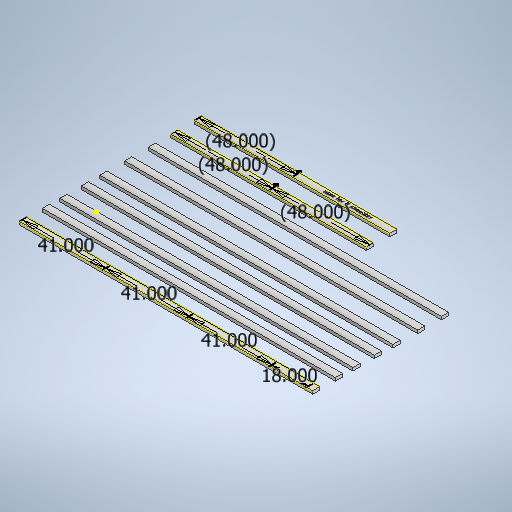
# Autodesk Inventor part: Lshoulder cuts
Saved by Autodesk Inventor 2026.1 (Build 301233000, 233)
## iProperties
Created: 2025-10-17
Part Number: Lshoulder cuts
Material: Generic
Document SubType Name: Modeling
Designer: jorda
Density: 1 g/cm^3
Appearance: Default
Author: jorda
Autodesk Inventor part; units mm, degrees
ref_plane "YZ Plane" through (0, 0, 0) normal (1, 0, 0) x (0, 1, 0)
ref_plane "XZ Plane" through (0, 0, 0) normal (0, 1, 0) x (-1, 0, 0)
ref_plane "XY Plane" through (0, 0, 0) normal (0, 0, 1) x (1, 0, 0)
sketch "Sketch1" plane through (0, 0, 0) normal (0, 1, 0) x (-1, 0, 0)
  line L0 (385.9062, 574.5992) -> (-3271.6938, 574.5992)
  line L1 (-3271.6938, 574.5992) -> (-3271.6938, 485.6992)
  line L2 (-3271.6938, 485.6992) -> (385.9062, 485.6992)
  line L3 (385.9062, 485.6992) -> (385.9062, 574.5992)
  line L4 (385.9062, 290.8577) -> (-3271.6938, 290.8577)
  line L5 (-3271.6938, 290.8577) -> (-3271.6938, 201.9577)
  line L6 (-3271.6938, 201.9577) -> (385.9062, 201.9577)
  line L7 (385.9062, 201.9577) -> (385.9062, 290.8577)
  line L8 (385.9062, 72.812) -> (-3271.6938, 72.812)
  line L9 (-3271.6938, 72.812) -> (-3271.6938, -16.088)
  line L10 (-3271.6938, -16.088) -> (385.9062, -16.088)
  line L11 (385.9062, -16.088) -> (385.9062, 72.812)
  line L12 (385.9062, -194.7435) -> (-3271.6938, -194.7435)
  line L13 (-3271.6938, -194.7435) -> (-3271.6938, -283.6435)
  line L14 (-3271.6938, -283.6435) -> (385.9062, -283.6435)
  line L15 (385.9062, -283.6435) -> (385.9062, -194.7435)
  line L16 (385.9062, -426.6687) -> (-3271.6938, -426.6687)
  line L17 (-3271.6938, -426.6687) -> (-3271.6938, -515.5687)
  line L18 (-3271.6938, -515.5687) -> (385.9062, -515.5687)
  line L19 (385.9062, -515.5687) -> (385.9062, -426.6687)
  line L20 (385.9062, -736.3666) -> (-3271.6938, -736.3666)
  line L21 (-3271.6938, -736.3666) -> (-3271.6938, -825.2666)
  line L22 (-3271.6938, -825.2666) -> (385.9062, -825.2666)
  line L23 (385.9062, -825.2666) -> (385.9062, -736.3666)
  line L24 (385.9062, -1031.6599) -> (-3271.6938, -1031.6599)
  line L25 (-3271.6938, -1031.6599) -> (-3271.6938, -1120.5599)
  line L26 (-3271.6938, -1120.5599) -> (385.9062, -1120.5599)
  line L27 (385.9062, -1120.5599) -> (385.9062, -1031.6599)
  line L28 (385.9062, -1312.5487) -> (-2052.4938, -1312.5487)
  line L29 (-2052.4938, -1312.5487) -> (-2052.4938, -1401.4487)
  line L30 (-2052.4938, -1401.4487) -> (385.9062, -1401.4487)
  line L31 (385.9062, -1401.4487) -> (385.9062, -1312.5487)
  line L32 (385.9062, -1607.8421) -> (-2052.4938, -1607.8421)
  line L33 (-2052.4938, -1607.8421) -> (-2052.4938, -1696.7421)
  line L34 (-2052.4938, -1696.7421) -> (385.9062, -1696.7421)
  line L35 (385.9062, -1696.7421) -> (385.9062, -1607.8421)
  point P0 (0, 0)
  constraints: 72 end point, 18 parallel, 9 horizontal, 9 perpendicular, 1 point on line
extrude "Extrusion1" add sketch "Sketch1" along normal blind 38.1
sketch "Sketch2" plane through (0, 38.1, 0) normal (0, 1, 0) x (1, 0, 0)
  line L0 (-385.9062, -574.5992) -> (3271.6938, -574.5992) projected
  line L1 (3271.6938, -485.6992) -> (-385.9062, -485.6992) projected
  line L2 (-385.9062, -574.5992) -> (655.4938, -574.5992)
  line L3 (655.4938, -574.5992) -> (655.4938, -485.6992)
  line L4 (655.4938, -485.6992) -> (-385.9062, -485.6992)
  line L5 (-385.9062, -485.6992) -> (-385.9062, -574.5992)
  line L6 (655.4938, -574.5992) -> (1696.8938, -574.5992)
  line L7 (1696.8938, -574.5992) -> (1696.8938, -485.6992)
  line L8 (1696.8938, -485.6992) -> (655.4938, -485.6992)
  line L9 (655.4938, -485.6992) -> (655.4938, -574.5992)
  line L10 (1696.8938, -574.5992) -> (2738.2938, -574.5992)
  line L11 (2738.2938, -574.5992) -> (2738.2938, -485.6992)
  line L12 (2738.2938, -485.6992) -> (1696.8938, -485.6992)
  line L13 (1696.8938, -485.6992) -> (1696.8938, -574.5992)
  line L14 (2738.2938, -574.5992) -> (3195.4938, -574.5992)
  line L15 (3195.4938, -574.5992) -> (3195.4938, -485.6992)
  line L16 (3195.4938, -485.6992) -> (2738.2938, -485.6992)
  line L17 (2738.2938, -485.6992) -> (2738.2938, -574.5992)
  point P0 (0, 0)
  dimension "d14" = 1041.4
  dimension "d15" = 1041.4
  dimension "d16" = 1041.4
  dimension "d17" = 457.2
  constraints: 32 end point, 8 parallel, 4 horizontal, 4 perpendicular, 4 point on line
  measures "d14" distance of L4.end L3.end
  measures "d15" distance of L8.end L7.end
  measures "d16" distance of L12.end L11.end
  measures "d17" distance of L16.end L15.end
sketch "Sketch3" plane through (0, 38.1, 0) normal (0, 1, 0) x (1, 0, 0)
  point P0 (0, 0)
sketch "Sketch4" plane through (0, 38.1, 0) normal (0, 1, 0) x (1, 0, 0)
  line L0 (-385.9062, 1312.5487) -> (2052.4938, 1312.5487) projected
  line L1 (-385.9062, 1312.5487) -> (833.2938, 1312.5487)
  line L2 (833.2938, 1312.5487) -> (744.3938, 1312.5487)
  line L3 (833.2938, 1312.5487) -> (833.2938, 1401.4487)
  line L4 (2052.4938, 1401.4487) -> (-385.9062, 1401.4487) projected
  line L5 (-385.9062, 1607.8421) -> (2052.4938, 1607.8421) projected
  line L6 (2052.4938, 1696.7421) -> (-385.9062, 1696.7421) projected
  line L7 (-385.9062, 1607.8421) -> (833.2938, 1607.8421)
  line L8 (833.2938, 1607.8421) -> (833.2938, 1696.7421)
  line L9 (833.2938, 1696.7421) -> (-385.9062, 1696.7421)
  line L10 (-385.9062, 1696.7421) -> (-385.9062, 1607.8421)
  line L11 (1180.5013, 1687.0985) -> (2076.0674, 1687.0985) construction
  line L12 (2076.0674, 1687.0985) -> (2076.0674, 1614.1334) construction
  line L13 (2076.0674, 1614.1334) -> (1180.5013, 1614.1334) construction
  line L14 (1180.5013, 1614.1334) -> (1180.5013, 1687.0985) construction
  point P0 (0, 0)
  dimension "d20" = 1219.2
  dimension "d21" = 1219.2
  dimension "d22" = 1219.2
  constraints: 14 end point, 6 midpoint, 2 parallel, 1 horizontal, 1 perpendicular, 1 point on line, 2 other
  measures "d20" distance of L4.end point (833.294, 1401.449)
  measures "d21" distance of L4.start point (833.294, 1401.449)
  measures "d22" distance of point (833.294, 1696.742) L6.end
body "Solid1"
